Spur Gear 10 teeth (16)-dup (Autodesk Fusion 360 design; units mm, degrees)
description: Spur Gear; Module: 1.27; Num Teeth: 10; Pressure Angle: 20.0; Backlash: 0.00 mm
part number: 2026-06-06-03-03-36-066
Autodesk Fusion 360 part; units mm, degrees
(part 1 of 2)
sketch "Base Circle" plane through (0, 0, 0) normal (0, 0, 1) x (1, 0, 0)
  circle A0 centre (0, 0) radius 4.8806
  circle A1 centre (0, 0) radius 2.5
extrude "Extrude1" add sketch "Base Circle" along normal blind 1
sketch "Gear Tooth" plane through (0, 0, 0) normal (0, 0, 1) x (1, 0, 0)
  spline S0 degree 5 poles (5.879, -1.0212) (5.8838, -1.022) (5.8935, -1.0235) (5.908, -1.0253) (5.9275, -1.0267) (5.952, -1.0272) (5.9766, -1.0267) (6.0013, -1.0257) (6.026, -1.0244) (6.0508, -1.0228) (6.0756, -1.021) (6.1004, -1.0189) (6.1253, -1.0165) (6.1502, -1.0135) (6.1752, -1.0101) (6.2001, -1.0063) (6.2251, -1.002) (6.2502, -0.9975) (6.2752, -0.9927) (6.3003, -0.9876) (6.3253, -0.9823) (6.3504, -0.9767) (6.3755, -0.9708) (6.4006, -0.9646) (6.4257, -0.9581) (6.4508, -0.9513) (6.4759, -0.9442) (6.501, -0.9369) (6.5261, -0.9293) (6.5512, -0.9215) (6.5763, -0.9134) (6.6014, -0.9051) (6.6265, -0.8965) (6.6516, -0.8877) (6.6767, -0.8786) (6.7018, -0.8693) (6.7268, -0.8598) (6.7519, -0.85) (6.7769, -0.84) (6.8019, -0.8297) (6.8269, -0.8193) (6.8519, -0.8086) (6.8768, -0.7977) (6.9017, -0.7865) (6.9267, -0.7752) (6.9515, -0.7636) (6.9764, -0.7518) (7.0012, -0.7398) (7.0261, -0.7275) (7.0508, -0.7151) (7.0756, -0.7025) (7.1003, -0.6896) (7.125, -0.6765) (7.1497, -0.6632) (7.1743, -0.6498) (7.1989, -0.6361) (7.2235, -0.6222) (7.248, -0.6081) (7.2725, -0.5938) (7.2969, -0.5793) (7.3213, -0.5646) (7.3457, -0.5497) (7.37, -0.5346) (7.3943, -0.5193) (7.4186, -0.5038) (7.4428, -0.4882) (7.4669, -0.4723) (7.491, -0.4562) (7.5151, -0.44) (7.5391, -0.4236) (7.5631, -0.4069) (7.5822, -0.3935) (7.5966, -0.3833) (7.6061, -0.3765) (7.6109, -0.373) knots 0 0 0 0 0 0 0.01428571 0.02857143 0.04285714 0.05714286 0.07142857 0.08571429 0.1 0.11428571 0.12857143 0.14285714 0.15714286 0.17142857 0.18571429 0.2 0.21428571 0.22857143 0.24285714 0.25714286 0.27142857 0.28571429 0.3 0.31428571 0.32857143 0.34285714 0.35714286 0.37142857 0.38571429 0.4 0.41428571 0.42857143 0.44285714 0.45714286 0.47142857 0.48571429 0.5 0.51428571 0.52857143 0.54285714 0.55714286 0.57142857 0.58571429 0.6 0.61428571 0.62857143 0.64285714 0.65714286 0.67142857 0.68571429 0.7 0.71428571 0.72857143 0.74285714 0.75714286 0.77142857 0.78571429 0.8 0.81428571 0.82857143 0.84285714 0.85714286 0.87142857 0.88571429 0.9 0.91428571 0.92857143 0.94285714 0.95714286 0.97142857 0.98571429 1 1 1 1 1 1
  spline S1 degree 5 poles (5.879, 1.0212) (5.8838, 1.022) (5.8935, 1.0235) (5.908, 1.0253) (5.9275, 1.0267) (5.952, 1.0272) (5.9766, 1.0267) (6.0013, 1.0257) (6.026, 1.0244) (6.0508, 1.0228) (6.0756, 1.021) (6.1004, 1.0189) (6.1253, 1.0165) (6.1502, 1.0135) (6.1752, 1.0101) (6.2001, 1.0063) (6.2251, 1.002) (6.2502, 0.9975) (6.2752, 0.9927) (6.3003, 0.9876) (6.3253, 0.9823) (6.3504, 0.9767) (6.3755, 0.9708) (6.4006, 0.9646) (6.4257, 0.9581) (6.4508, 0.9513) (6.4759, 0.9442) (6.501, 0.9369) (6.5261, 0.9293) (6.5512, 0.9215) (6.5763, 0.9134) (6.6014, 0.9051) (6.6265, 0.8965) (6.6516, 0.8877) (6.6767, 0.8786) (6.7018, 0.8693) (6.7268, 0.8598) (6.7519, 0.85) (6.7769, 0.84) (6.8019, 0.8297) (6.8269, 0.8193) (6.8519, 0.8086) (6.8768, 0.7977) (6.9017, 0.7865) (6.9267, 0.7752) (6.9515, 0.7636) (6.9764, 0.7518) (7.0012, 0.7398) (7.0261, 0.7275) (7.0508, 0.7151) (7.0756, 0.7025) (7.1003, 0.6896) (7.125, 0.6765) (7.1497, 0.6632) (7.1743, 0.6498) (7.1989, 0.6361) (7.2235, 0.6222) (7.248, 0.6081) (7.2725, 0.5938) (7.2969, 0.5793) (7.3213, 0.5646) (7.3457, 0.5497) (7.37, 0.5346) (7.3943, 0.5193) (7.4186, 0.5038) (7.4428, 0.4882) (7.4669, 0.4723) (7.491, 0.4562) (7.5151, 0.44) (7.5391, 0.4236) (7.5631, 0.4069) (7.5822, 0.3935) (7.5966, 0.3833) (7.6061, 0.3765) (7.6109, 0.373) knots 0 0 0 0 0 0 0.01428571 0.02857143 0.04285714 0.05714286 0.07142857 0.08571429 0.1 0.11428571 0.12857143 0.14285714 0.15714286 0.17142857 0.18571429 0.2 0.21428571 0.22857143 0.24285714 0.25714286 0.27142857 0.28571429 0.3 0.31428571 0.32857143 0.34285714 0.35714286 0.37142857 0.38571429 0.4 0.41428571 0.42857143 0.44285714 0.45714286 0.47142857 0.48571429 0.5 0.51428571 0.52857143 0.54285714 0.55714286 0.57142857 0.58571429 0.6 0.61428571 0.62857143 0.64285714 0.65714286 0.67142857 0.68571429 0.7 0.71428571 0.72857143 0.74285714 0.75714286 0.77142857 0.78571429 0.8 0.81428571 0.82857143 0.84285714 0.85714286 0.87142857 0.88571429 0.9 0.91428571 0.92857143 0.94285714 0.95714286 0.97142857 0.98571429 1 1 1 1 1 1
  arc A0 (7.6109, -0.373) -> (7.6109, 0.373) centre (0, 0) ccw
  line L0 (4.7988, -0.8335) -> (5.879, -1.0212)
  line L1 (4.7988, 0.8335) -> (5.879, 1.0212)
  line L2 (4.7988, -0.8335) -> (4.7988, 0.8335)
  point P0 (5.998, -1.0258)
  point P1 (6.1192, -1.017)
  point P2 (6.2418, -0.999)
  point P3 (6.3654, -0.9731)
  point P4 (6.4896, -0.9402)
  point P5 (6.6144, -0.9006)
  point P6 (6.7395, -0.8548)
  point P7 (6.8648, -0.8029)
  point P8 (6.9901, -0.7452)
  point P9 (7.1151, -0.6817)
  point P10 (7.2399, -0.6127)
  point P11 (7.3642, -0.5382)
  point P12 (7.4879, -0.4583)
  point P13 (5.998, 1.0258)
  point P14 (6.1192, 1.017)
  point P15 (6.2418, 0.999)
  point P16 (6.3654, 0.9731)
  point P17 (6.4896, 0.9402)
  point P18 (6.6144, 0.9006)
  point P19 (6.7395, 0.8548)
  point P20 (6.8648, 0.8029)
  point P21 (6.9901, 0.7452)
  point P22 (7.1151, 0.6817)
  point P23 (7.2399, 0.6127)
  point P24 (7.3642, 0.5382)
  point P25 (7.4879, 0.4583)
extrude "Extrude2" add sketch "Gear Tooth" along normal blind 1
fillet "Fillet1" radius 0.2 2 edges at (4.8086, -0.8353, 0.5) (4.8086, 0.8353, 0.5)
pattern_circular "C-Pattern1" count 10 over 360 about axis through (0, 0, 0) along (0, 0, 1) of "Extrude2", "Fillet1"
sketch "Diametrial Pitch Circle" plane through (0, 0, 0) normal (0, 0, 1) x (1, 0, 0)
  circle A0 centre (0, 0) radius 6.35 construction
extrude "Extrude3" add 1 faces at (4.0508, 0, 0) along direction (0, 0, -1) blind 2
extrude "Extrude4" add 1 faces at (4.0508, 0, 1) along direction (0, 0, 1) blind 3
sketch "Sketch4" plane through (0, 0, 4) normal (0, 0, 1) x (1, 0, 0)
  arc A0 (4.4625, -1.9766) -> (4.772, -1.0239) centre (0, 0) ccw
  arc A1 (5.0018, -0.8688) -> (4.772, -1.0239) centre (4.9675, -1.0659) ccw
  line L0 (5.0018, -0.8688) -> (5.879, -1.0212)
  spline S0 degree 5 poles (5.879, -1.0212) (5.8838, -1.022) (5.8935, -1.0235) (5.908, -1.0253) (5.9275, -1.0267) (5.952, -1.0272) (5.9766, -1.0267) (6.0013, -1.0257) (6.026, -1.0244) (6.0508, -1.0228) (6.0756, -1.021) (6.1004, -1.0189) (6.1253, -1.0165) (6.1502, -1.0135) (6.1752, -1.0101) (6.2001, -1.0063) (6.2251, -1.002) (6.2502, -0.9975) (6.2752, -0.9927) (6.3003, -0.9876) (6.3253, -0.9823) (6.3504, -0.9767) (6.3755, -0.9708) (6.4006, -0.9646) (6.4257, -0.9581) (6.4508, -0.9513) (6.4759, -0.9442) (6.501, -0.9369) (6.5261, -0.9293) (6.5512, -0.9215) (6.5763, -0.9134) (6.6014, -0.9051) (6.6265, -0.8965) (6.6516, -0.8877) (6.6767, -0.8786) (6.7018, -0.8693) (6.7268, -0.8598) (6.7519, -0.85) (6.7769, -0.84) (6.8019, -0.8297) (6.8269, -0.8193) (6.8519, -0.8086) (6.8768, -0.7977) (6.9017, -0.7865) (6.9267, -0.7752) (6.9515, -0.7636) (6.9764, -0.7518) (7.0012, -0.7398) (7.0261, -0.7275) (7.0508, -0.7151) (7.0756, -0.7025) (7.1003, -0.6896) (7.125, -0.6765) (7.1497, -0.6632) (7.1743, -0.6498) (7.1989, -0.6361) (7.2235, -0.6222) (7.248, -0.6081) (7.2725, -0.5938) (7.2969, -0.5793) (7.3213, -0.5646) (7.3457, -0.5497) (7.37, -0.5346) (7.3943, -0.5193) (7.4186, -0.5038) (7.4428, -0.4882) (7.4669, -0.4723) (7.491, -0.4562) (7.5151, -0.44) (7.5391, -0.4236) (7.5631, -0.4069) (7.5822, -0.3935) (7.5966, -0.3833) (7.6061, -0.3765) (7.6109, -0.373) knots 0 0 0 0 0 0 0.01428571 0.02857143 0.04285714 0.05714286 0.07142857 0.08571429 0.1 0.11428571 0.12857143 0.14285714 0.15714286 0.17142857 0.18571429 0.2 0.21428571 0.22857143 0.24285714 0.25714286 0.27142857 0.28571429 0.3 0.31428571 0.32857143 0.34285714 0.35714286 0.37142857 0.38571429 0.4 0.41428571 0.42857143 0.44285714 0.45714286 0.47142857 0.48571429 0.5 0.51428571 0.52857143 0.54285714 0.55714286 0.57142857 0.58571429 0.6 0.61428571 0.62857143 0.64285714 0.65714286 0.67142857 0.68571429 0.7 0.71428571 0.72857143 0.74285714 0.75714286 0.77142857 0.78571429 0.8 0.81428571 0.82857143 0.84285714 0.85714286 0.87142857 0.88571429 0.9 0.91428571 0.92857143 0.94285714 0.95714286 0.97142857 0.98571429 1 1 1 1 1 1
  arc A2 (7.6109, -0.373) -> (7.6109, 0.373) centre (0, 0) ccw
  spline S1 degree 5 poles (7.6109, 0.373) (7.6061, 0.3765) (7.5966, 0.3833) (7.5822, 0.3935) (7.5631, 0.4069) (7.5391, 0.4236) (7.5151, 0.44) (7.491, 0.4562) (7.4669, 0.4723) (7.4428, 0.4882) (7.4186, 0.5038) (7.3943, 0.5193) (7.37, 0.5346) (7.3457, 0.5497) (7.3213, 0.5646) (7.2969, 0.5793) (7.2725, 0.5938) (7.248, 0.6081) (7.2235, 0.6222) (7.1989, 0.6361) (7.1743, 0.6498) (7.1497, 0.6632) (7.125, 0.6765) (7.1003, 0.6896) (7.0756, 0.7025) (7.0508, 0.7151) (7.0261, 0.7275) (7.0012, 0.7398) (6.9764, 0.7518) (6.9515, 0.7636) (6.9267, 0.7752) (6.9017, 0.7865) (6.8768, 0.7977) (6.8519, 0.8086) (6.8269, 0.8193) (6.8019, 0.8297) (6.7769, 0.84) (6.7519, 0.85) (6.7268, 0.8598) (6.7018, 0.8693) (6.6767, 0.8786) (6.6516, 0.8877) (6.6265, 0.8965) (6.6014, 0.9051) (6.5763, 0.9134) (6.5512, 0.9215) (6.5261, 0.9293) (6.501, 0.9369) (6.4759, 0.9442) (6.4508, 0.9513) (6.4257, 0.9581) (6.4006, 0.9646) (6.3755, 0.9708) (6.3504, 0.9767) (6.3253, 0.9823) (6.3003, 0.9876) (6.2752, 0.9927) (6.2502, 0.9975) (6.2251, 1.002) (6.2001, 1.0063) (6.1752, 1.0101) (6.1502, 1.0135) (6.1253, 1.0165) (6.1004, 1.0189) (6.0756, 1.021) (6.0508, 1.0228) (6.026, 1.0244) (6.0013, 1.0257) (5.9766, 1.0267) (5.952, 1.0272) (5.9275, 1.0267) (5.908, 1.0253) (5.8935, 1.0235) (5.8838, 1.022) (5.879, 1.0212) knots -1 -1 -1 -1 -1 -1 -0.98571429 -0.97142857 -0.95714286 -0.94285714 -0.92857143 -0.91428571 -0.9 -0.88571429 -0.87142857 -0.85714286 -0.84285714 -0.82857143 -0.81428571 -0.8 -0.78571429 -0.77142857 -0.75714286 -0.74285714 -0.72857143 -0.71428571 -0.7 -0.68571429 -0.67142857 -0.65714286 -0.64285714 -0.62857143 -0.61428571 -0.6 -0.58571429 -0.57142857 -0.55714286 -0.54285714 -0.52857143 -0.51428571 -0.5 -0.48571429 -0.47142857 -0.45714286 -0.44285714 -0.42857143 -0.41428571 -0.4 -0.38571429 -0.37142857 -0.35714286 -0.34285714 -0.32857143 -0.31428571 -0.3 -0.28571429 -0.27142857 -0.25714286 -0.24285714 -0.22857143 -0.21428571 -0.2 -0.18571429 -0.17142857 -0.15714286 -0.14285714 -0.12857143 -0.11428571 -0.1 -0.08571429 -0.07142857 -0.05714286 -0.04285714 -0.02857143 -0.01428571 0 0 0 0 0 0
  line L1 (5.879, 1.0212) -> (5.0018, 0.8688)
  arc A3 (4.772, 1.0239) -> (5.0018, 0.8688) centre (4.9675, 1.0659) ccw
  arc A4 (4.772, 1.0239) -> (4.4625, 1.9766) centre (0, 0) ccw
  arc A5 (4.5572, 2.2371) -> (4.4625, 1.9766) centre (4.6453, 2.0576) ccw
  line L2 (4.5572, 2.2371) -> (5.3565, 2.6294)
  spline S2 degree 5 poles (5.3565, 2.6294) (5.3609, 2.6316) (5.3696, 2.6361) (5.3824, 2.6432) (5.3989, 2.6535) (5.419, 2.6675) (5.4387, 2.6823) (5.458, 2.6976) (5.4773, 2.7133) (5.4964, 2.7291) (5.5154, 2.7451) (5.5343, 2.7614) (5.5529, 2.778) (5.5713, 2.7951) (5.5895, 2.8125) (5.6075, 2.8303) (5.6252, 2.8484) (5.6428, 2.8668) (5.6602, 2.8854) (5.6775, 2.9042) (5.6947, 2.9233) (5.7117, 2.9425) (5.7285, 2.9621) (5.7451, 2.9818) (5.7616, 3.0018) (5.7779, 3.0221) (5.7941, 3.0426) (5.8101, 3.0633) (5.826, 3.0842) (5.8417, 3.1052) (5.8572, 3.1265) (5.8727, 3.148) (5.8879, 3.1697) (5.903, 3.1916) (5.918, 3.2137) (5.9328, 3.2359) (5.9475, 3.2584) (5.962, 3.281) (5.9763, 3.3038) (5.9905, 3.3268) (6.0046, 3.3499) (6.0185, 3.3733) (6.0323, 3.3968) (6.0459, 3.4204) (6.0594, 3.4443) (6.0727, 3.4683) (6.0859, 3.4924) (6.099, 3.5167) (6.1118, 3.5412) (6.1246, 3.5658) (6.1372, 3.5906) (6.1496, 3.6156) (6.1619, 3.6407) (6.1741, 3.6659) (6.1861, 3.6913) (6.1979, 3.7168) (6.2096, 3.7425) (6.2212, 3.7683) (6.2326, 3.7943) (6.2438, 3.8204) (6.255, 3.8466) (6.2659, 3.873) (6.2767, 3.8995) (6.2874, 3.9261) (6.2979, 3.9529) (6.3083, 3.9798) (6.3185, 4.0069) (6.3286, 4.034) (6.3385, 4.0613) (6.3482, 4.0887) (6.3579, 4.1163) (6.3654, 4.1384) (6.371, 4.1551) (6.3747, 4.1662) (6.3766, 4.1718) knots 0 0 0 0 0 0 0.01428571 0.02857143 0.04285714 0.05714286 0.07142857 0.08571429 0.1 0.11428571 0.12857143 0.14285714 0.15714286 0.17142857 0.18571429 0.2 0.21428571 0.22857143 0.24285714 0.25714286 0.27142857 0.28571429 0.3 0.31428571 0.32857143 0.34285714 0.35714286 0.37142857 0.38571429 0.4 0.41428571 0.42857143 0.44285714 0.45714286 0.47142857 0.48571429 0.5 0.51428571 0.52857143 0.54285714 0.55714286 0.57142857 0.58571429 0.6 0.61428571 0.62857143 0.64285714 0.65714286 0.67142857 0.68571429 0.7 0.71428571 0.72857143 0.74285714 0.75714286 0.77142857 0.78571429 0.8 0.81428571 0.82857143 0.84285714 0.85714286 0.87142857 0.88571429 0.9 0.91428571 0.92857143 0.94285714 0.95714286 0.97142857 0.98571429 1 1 1 1 1 1
  arc A6 (6.3766, 4.1718) -> (5.938, 4.7754) centre (0, 0) ccw
  spline S3 degree 5 poles (5.938, 4.7754) (5.9322, 4.7753) (5.9204, 4.7752) (5.9029, 4.775) (5.8795, 4.7747) (5.8503, 4.774) (5.8212, 4.7732) (5.7922, 4.7722) (5.7633, 4.7711) (5.7344, 4.7697) (5.7056, 4.7682) (5.6769, 4.7664) (5.6483, 4.7645) (5.6197, 4.7624) (5.5912, 4.7602) (5.5628, 4.7577) (5.5345, 4.755) (5.5063, 4.7522) (5.4782, 4.7492) (5.4502, 4.746) (5.4222, 4.7426) (5.3944, 4.7391) (5.3666, 4.7353) (5.3389, 4.7314) (5.3114, 4.7272) (5.2839, 4.7229) (5.2566, 4.7184) (5.2293, 4.7137) (5.2021, 4.7088) (5.1751, 4.7038) (5.1481, 4.6985) (5.1213, 4.6931) (5.0946, 4.6874) (5.068, 4.6816) (5.0415, 4.6755) (5.0151, 4.6693) (4.9889, 4.6629) (4.9628, 4.6563) (4.9368, 4.6495) (4.9109, 4.6425) (4.8851, 4.6353) (4.8595, 4.6279) (4.834, 4.6203) (4.8087, 4.6124) (4.7835, 4.6044) (4.7584, 4.5962) (4.7335, 4.5878) (4.7088, 4.5791) (4.6841, 4.5703) (4.6597, 4.5613) (4.6354, 4.552) (4.6112, 4.5425) (4.5873, 4.5328) (4.5635, 4.5228) (4.5399, 4.5126) (4.5165, 4.5022) (4.4933, 4.4916) (4.4702, 4.4807) (4.4473, 4.4697) (4.4246, 4.4584) (4.4021, 4.4468) (4.3799, 4.4349) (4.358, 4.4227) (4.3364, 4.4101) (4.3151, 4.3972) (4.294, 4.384) (4.273, 4.3707) (4.2522, 4.3573) (4.2317, 4.3436) (4.2115, 4.3295) (4.192, 4.3147) (4.177, 4.3021) (4.1663, 4.2922) (4.1594, 4.2853) (4.156, 4.2818) knots -1 -1 -1 -1 -1 -1 -0.98571429 -0.97142857 -0.95714286 -0.94285714 -0.92857143 -0.91428571 -0.9 -0.88571429 -0.87142857 -0.85714286 -0.84285714 -0.82857143 -0.81428571 -0.8 -0.78571429 -0.77142857 -0.75714286 -0.74285714 -0.72857143 -0.71428571 -0.7 -0.68571429 -0.67142857 -0.65714286 -0.64285714 -0.62857143 -0.61428571 -0.6 -0.58571429 -0.57142857 -0.55714286 -0.54285714 -0.52857143 -0.51428571 -0.5 -0.48571429 -0.47142857 -0.45714286 -0.44285714 -0.42857143 -0.41428571 -0.4 -0.38571429 -0.37142857 -0.35714286 -0.34285714 -0.32857143 -0.31428571 -0.3 -0.28571429 -0.27142857 -0.25714286 -0.24285714 -0.22857143 -0.21428571 -0.2 -0.18571429 -0.17142857 -0.15714286 -0.14285714 -0.12857143 -0.11428571 -0.1 -0.08571429 -0.07142857 -0.05714286 -0.04285714 -0.02857143 -0.01428571 0 0 0 0 0 0
  line L3 (4.156, 4.2818) -> (3.5358, 3.6429)
  arc A7 (3.2588, 3.6333) -> (3.5358, 3.6429) centre (3.3923, 3.7821) ccw
  arc A8 (3.2588, 3.6333) -> (2.4484, 4.222) centre (0, 0) ccw
  arc A9 (2.3719, 4.4885) -> (2.4484, 4.222) centre (2.5487, 4.3951) ccw
  line L4 (2.3719, 4.4885) -> (2.7879, 5.2757)
  spline S4 degree 5 poles (2.7879, 5.2757) (2.7902, 5.28) (2.7946, 5.2888) (2.8008, 5.302) (2.8082, 5.3201) (2.8162, 5.3433) (2.8234, 5.3668) (2.83, 5.3906) (2.8364, 5.4145) (2.8426, 5.4386) (2.8485, 5.4627) (2.8542, 5.487) (2.8595, 5.5114) (2.8644, 5.536) (2.8689, 5.5608) (2.8729, 5.5857) (2.8767, 5.6108) (2.8801, 5.636) (2.8832, 5.6613) (2.8862, 5.6867) (2.8888, 5.7122) (2.8912, 5.7378) (2.8934, 5.7635) (2.8952, 5.7893) (2.8968, 5.8151) (2.8981, 5.8411) (2.8991, 5.8672) (2.8999, 5.8933) (2.9005, 5.9196) (2.9008, 5.9459) (2.9009, 5.9722) (2.9007, 5.9987) (2.9003, 6.0252) (2.8997, 6.0518) (2.8988, 6.0784) (2.8977, 6.1051) (2.8964, 6.1319) (2.8948, 6.1587) (2.893, 6.1856) (2.891, 6.2126) (2.8888, 6.2396) (2.8863, 6.2666) (2.8837, 6.2937) (2.8808, 6.3209) (2.8777, 6.3481) (2.8744, 6.3753) (2.8708, 6.4026) (2.8671, 6.43) (2.8631, 6.4574) (2.8589, 6.4848) (2.8546, 6.5122) (2.85, 6.5397) (2.8452, 6.5672) (2.8402, 6.5948) (2.8349, 6.6224) (2.8295, 6.65) (2.8239, 6.6777) (2.8181, 6.7053) (2.8121, 6.7331) (2.8058, 6.7608) (2.7994, 6.7885) (2.7928, 6.8163) (2.7859, 6.8441) (2.7789, 6.872) (2.7717, 6.8998) (2.7642, 6.9277) (2.7566, 6.9555) (2.7488, 6.9834) (2.7408, 7.0113) (2.7325, 7.0392) (2.7241, 7.0672) (2.7172, 7.0895) (2.712, 7.1063) (2.7085, 7.1175) (2.7067, 7.1231) knots 0 0 0 0 0 0 0.01428571 0.02857143 0.04285714 0.05714286 0.07142857 0.08571429 0.1 0.11428571 0.12857143 0.14285714 0.15714286 0.17142857 0.18571429 0.2 0.21428571 0.22857143 0.24285714 0.25714286 0.27142857 0.28571429 0.3 0.31428571 0.32857143 0.34285714 0.35714286 0.37142857 0.38571429 0.4 0.41428571 0.42857143 0.44285714 0.45714286 0.47142857 0.48571429 0.5 0.51428571 0.52857143 0.54285714 0.55714286 0.57142857 0.58571429 0.6 0.61428571 0.62857143 0.64285714 0.65714286 0.67142857 0.68571429 0.7 0.71428571 0.72857143 0.74285714 0.75714286 0.77142857 0.78571429 0.8 0.81428571 0.82857143 0.84285714 0.85714286 0.87142857 0.88571429 0.9 0.91428571 0.92857143 0.94285714 0.95714286 0.97142857 0.98571429 1 1 1 1 1 1
  arc A10 (2.7067, 7.1231) -> (1.9971, 7.3536) centre (0, 0) ccw
  spline S5 degree 5 poles (1.9971, 7.3536) (1.9924, 7.3502) (1.9829, 7.3432) (1.9688, 7.3327) (1.9501, 7.3187) (1.9269, 7.301) (1.9038, 7.2833) (1.8809, 7.2654) (1.8582, 7.2474) (1.8357, 7.2294) (1.8133, 7.2112) (1.7911, 7.1929) (1.769, 7.1745) (1.7471, 7.1561) (1.7255, 7.1375) (1.7039, 7.1188) (1.6826, 7.1) (1.6614, 7.0812) (1.6404, 7.0622) (1.6196, 7.0431) (1.599, 7.024) (1.5786, 7.0047) (1.5583, 6.9854) (1.5383, 6.9659) (1.5184, 6.9464) (1.4987, 6.9267) (1.4792, 6.907) (1.4599, 6.8872) (1.4408, 6.8673) (1.4219, 6.8473) (1.4032, 6.8272) (1.3847, 6.807) (1.3664, 6.7867) (1.3483, 6.7664) (1.3305, 6.7459) (1.3128, 6.7254) (1.2953, 6.7048) (1.2781, 6.6841) (1.261, 6.6633) (1.2442, 6.6424) (1.2276, 6.6214) (1.2112, 6.6004) (1.1951, 6.5792) (1.1792, 6.558) (1.1635, 6.5367) (1.1481, 6.5153) (1.1329, 6.4939) (1.1179, 6.4723) (1.1032, 6.4507) (1.0887, 6.429) (1.0745, 6.4072) (1.0605, 6.3854) (1.0469, 6.3634) (1.0335, 6.3414) (1.0204, 6.3193) (1.0076, 6.2971) (0.995, 6.2748) (0.9827, 6.2525) (0.9707, 6.2301) (0.9589, 6.2076) (0.9476, 6.1851) (0.9366, 6.1624) (0.9261, 6.1396) (0.9161, 6.1167) (0.9064, 6.0937) (0.897, 6.0707) (0.8879, 6.0476) (0.879, 6.0245) (0.8704, 6.0014) (0.8623, 5.9781) (0.8552, 5.9547) (0.8506, 5.9357) (0.8478, 5.9213) (0.8462, 5.9117) (0.8455, 5.9068) knots -1 -1 -1 -1 -1 -1 -0.98571429 -0.97142857 -0.95714286 -0.94285714 -0.92857143 -0.91428571 -0.9 -0.88571429 -0.87142857 -0.85714286 -0.84285714 -0.82857143 -0.81428571 -0.8 -0.78571429 -0.77142857 -0.75714286 -0.74285714 -0.72857143 -0.71428571 -0.7 -0.68571429 -0.67142857 -0.65714286 -0.64285714 -0.62857143 -0.61428571 -0.6 -0.58571429 -0.57142857 -0.55714286 -0.54285714 -0.52857143 -0.51428571 -0.5 -0.48571429 -0.47142857 -0.45714286 -0.44285714 -0.42857143 -0.41428571 -0.4 -0.38571429 -0.37142857 -0.35714286 -0.34285714 -0.32857143 -0.31428571 -0.3 -0.28571429 -0.27142857 -0.25714286 -0.24285714 -0.22857143 -0.21428571 -0.2 -0.18571429 -0.17142857 -0.15714286 -0.14285714 -0.12857143 -0.11428571 -0.1 -0.08571429 -0.07142857 -0.05714286 -0.04285714 -0.02857143 -0.01428571 0 0 0 0 0 0
  line L5 (0.8455, 5.9068) -> (0.7193, 5.0254)
  arc A11 (0.5008, 4.8548) -> (0.7193, 5.0254) centre (0.5214, 5.0538) ccw
  arc A12 (0.5008, 4.8548) -> (-0.5008, 4.8548) centre (0, 0) ccw
  arc A13 (-0.7193, 5.0254) -> (-0.5008, 4.8548) centre (-0.5214, 5.0538) ccw
  line L6 (-0.7193, 5.0254) -> (-0.8455, 5.9068)
  spline S6 degree 5 poles (-0.8455, 5.9068) (-0.8462, 5.9117) (-0.8478, 5.9213) (-0.8506, 5.9357) (-0.8552, 5.9547) (-0.8623, 5.9781) (-0.8704, 6.0014) (-0.879, 6.0245) (-0.8879, 6.0476) (-0.897, 6.0707) (-0.9064, 6.0937) (-0.9161, 6.1167) (-0.9261, 6.1396) (-0.9366, 6.1624) (-0.9476, 6.1851) (-0.9589, 6.2076) (-0.9707, 6.2301) (-0.9827, 6.2525) (-0.995, 6.2748) (-1.0076, 6.2971) (-1.0204, 6.3193) (-1.0335, 6.3414) (-1.0469, 6.3634) (-1.0605, 6.3854) (-1.0745, 6.4072) (-1.0887, 6.429) (-1.1032, 6.4507) (-1.1179, 6.4723) (-1.1329, 6.4939) (-1.1481, 6.5153) (-1.1635, 6.5367) (-1.1792, 6.558) (-1.1951, 6.5792) (-1.2112, 6.6004) (-1.2276, 6.6214) (-1.2442, 6.6424) (-1.261, 6.6633) (-1.2781, 6.6841) (-1.2953, 6.7048) (-1.3128, 6.7254) (-1.3305, 6.7459) (-1.3483, 6.7664) (-1.3664, 6.7867) (-1.3847, 6.807) (-1.4032, 6.8272) (-1.4219, 6.8473) (-1.4408, 6.8673) (-1.4599, 6.8872) (-1.4792, 6.907) (-1.4987, 6.9267) (-1.5184, 6.9464) (-1.5383, 6.9659) (-1.5583, 6.9854) (-1.5786, 7.0047) (-1.599, 7.024) (-1.6196, 7.0431) (-1.6404, 7.0622) (-1.6614, 7.0812) (-1.6826, 7.1) (-1.7039, 7.1188) (-1.7255, 7.1375) (-1.7471, 7.1561) (-1.769, 7.1745) (-1.7911, 7.1929) (-1.8133, 7.2112) (-1.8357, 7.2294) (-1.8582, 7.2474) (-1.8809, 7.2654) (-1.9038, 7.2833) (-1.9269, 7.301) (-1.9501, 7.3187) (-1.9688, 7.3327) (-1.9829, 7.3432) (-1.9924, 7.3502) (-1.9971, 7.3536) knots 0 0 0 0 0 0 0.01428571 0.02857143 0.04285714 0.05714286 0.07142857 0.08571429 0.1 0.11428571 0.12857143 0.14285714 0.15714286 0.17142857 0.18571429 0.2 0.21428571 0.22857143 0.24285714 0.25714286 0.27142857 0.28571429 0.3 0.31428571 0.32857143 0.34285714 0.35714286 0.37142857 0.38571429 0.4 0.41428571 0.42857143 0.44285714 0.45714286 0.47142857 0.48571429 0.5 0.51428571 0.52857143 0.54285714 0.55714286 0.57142857 0.58571429 0.6 0.61428571 0.62857143 0.64285714 0.65714286 0.67142857 0.68571429 0.7 0.71428571 0.72857143 0.74285714 0.75714286 0.77142857 0.78571429 0.8 0.81428571 0.82857143 0.84285714 0.85714286 0.87142857 0.88571429 0.9 0.91428571 0.92857143 0.94285714 0.95714286 0.97142857 0.98571429 1 1 1 1 1 1
  arc A14 (-1.9971, 7.3536) -> (-2.7067, 7.1231) centre (0, 0) ccw
  spline S7 degree 5 poles (-2.7067, 7.1231) (-2.7085, 7.1175) (-2.712, 7.1063) (-2.7172, 7.0895) (-2.7241, 7.0672) (-2.7325, 7.0392) (-2.7408, 7.0113) (-2.7488, 6.9834) (-2.7566, 6.9555) (-2.7642, 6.9277) (-2.7717, 6.8998) (-2.7789, 6.872) (-2.7859, 6.8441) (-2.7928, 6.8163) (-2.7994, 6.7885) (-2.8058, 6.7608) (-2.8121, 6.7331) (-2.8181, 6.7053) (-2.8239, 6.6777) (-2.8295, 6.65) (-2.8349, 6.6224) (-2.8402, 6.5948) (-2.8452, 6.5672) (-2.85, 6.5397) (-2.8546, 6.5122) (-2.8589, 6.4848) (-2.8631, 6.4574) (-2.8671, 6.43) (-2.8708, 6.4026) (-2.8744, 6.3753) (-2.8777, 6.3481) (-2.8808, 6.3209) (-2.8837, 6.2937) (-2.8863, 6.2666) (-2.8888, 6.2396) (-2.891, 6.2126) (-2.893, 6.1856) (-2.8948, 6.1587) (-2.8964, 6.1319) (-2.8977, 6.1051) (-2.8988, 6.0784) (-2.8997, 6.0518) (-2.9003, 6.0252) (-2.9007, 5.9987) (-2.9009, 5.9722) (-2.9008, 5.9459) (-2.9005, 5.9196) (-2.8999, 5.8933) (-2.8991, 5.8672) (-2.8981, 5.8411) (-2.8968, 5.8151) (-2.8952, 5.7893) (-2.8934, 5.7635) (-2.8912, 5.7378) (-2.8888, 5.7122) (-2.8862, 5.6867) (-2.8832, 5.6613) (-2.8801, 5.636) (-2.8767, 5.6108) (-2.8729, 5.5857) (-2.8689, 5.5608) (-2.8644, 5.536) (-2.8595, 5.5114) (-2.8542, 5.487) (-2.8485, 5.4627) (-2.8426, 5.4386) (-2.8364, 5.4145) (-2.83, 5.3906) (-2.8234, 5.3668) (-2.8162, 5.3433) (-2.8082, 5.3201) (-2.8008, 5.302) (-2.7946, 5.2888) (-2.7902, 5.28) (-2.7879, 5.2757) knots -1 -1 -1 -1 -1 -1 -0.98571429 -0.97142857 -0.95714286 -0.94285714 -0.92857143 -0.91428571 -0.9 -0.88571429 -0.87142857 -0.85714286 -0.84285714 -0.82857143 -0.81428571 -0.8 -0.78571429 -0.77142857 -0.75714286 -0.74285714 -0.72857143 -0.71428571 -0.7 -0.68571429 -0.67142857 -0.65714286 -0.64285714 -0.62857143 -0.61428571 -0.6 -0.58571429 -0.57142857 -0.55714286 -0.54285714 -0.52857143 -0.51428571 -0.5 -0.48571429 -0.47142857 -0.45714286 -0.44285714 -0.42857143 -0.41428571 -0.4 -0.38571429 -0.37142857 -0.35714286 -0.34285714 -0.32857143 -0.31428571 -0.3 -0.28571429 -0.27142857 -0.25714286 -0.24285714 -0.22857143 -0.21428571 -0.2 -0.18571429 -0.17142857 -0.15714286 -0.14285714 -0.12857143 -0.11428571 -0.1 -0.08571429 -0.07142857 -0.05714286 -0.04285714 -0.02857143 -0.01428571 0 0 0 0 0 0
  line L7 (-2.7879, 5.2757) -> (-2.3719, 4.4885)
  arc A15 (-2.4484, 4.222) -> (-2.3719, 4.4885) centre (-2.5487, 4.3951) ccw
  arc A16 (-2.4484, 4.222) -> (-3.2588, 3.6333) centre (0, 0) ccw
  arc A17 (-3.5358, 3.6429) -> (-3.2588, 3.6333) centre (-3.3923, 3.7821) ccw
  line L8 (-3.5358, 3.6429) -> (-4.156, 4.2818)
  spline S8 degree 5 poles (-4.156, 4.2818) (-4.1594, 4.2853) (-4.1663, 4.2922) (-4.177, 4.3021) (-4.192, 4.3147) (-4.2115, 4.3295) (-4.2317, 4.3436) (-4.2522, 4.3573) (-4.273, 4.3707) (-4.294, 4.384) (-4.3151, 4.3972) (-4.3364, 4.4101) (-4.358, 4.4227) (-4.3799, 4.4349) (-4.4021, 4.4468) (-4.4246, 4.4584) (-4.4473, 4.4697) (-4.4702, 4.4807) (-4.4933, 4.4916) (-4.5165, 4.5022) (-4.5399, 4.5126) (-4.5635, 4.5228) (-4.5873, 4.5328) (-4.6112, 4.5425) (-4.6354, 4.552) (-4.6597, 4.5613) (-4.6841, 4.5703) (-4.7088, 4.5791) (-4.7335, 4.5878) (-4.7584, 4.5962) (-4.7835, 4.6044) (-4.8087, 4.6124) (-4.834, 4.6203) (-4.8595, 4.6279) (-4.8851, 4.6353) (-4.9109, 4.6425) (-4.9368, 4.6495) (-4.9628, 4.6563) (-4.9889, 4.6629) (-5.0151, 4.6693) (-5.0415, 4.6755) (-5.068, 4.6816) (-5.0946, 4.6874) (-5.1213, 4.6931) (-5.1481, 4.6985) (-5.1751, 4.7038) (-5.2021, 4.7088) (-5.2293, 4.7137) (-5.2566, 4.7184) (-5.2839, 4.7229) (-5.3114, 4.7272) (-5.3389, 4.7314) (-5.3666, 4.7353) (-5.3944, 4.7391) (-5.4222, 4.7426) (-5.4502, 4.746) (-5.4782, 4.7492) (-5.5063, 4.7522) (-5.5345, 4.755) (-5.5628, 4.7577) (-5.5912, 4.7602) (-5.6197, 4.7624) (-5.6483, 4.7645) (-5.6769, 4.7664) (-5.7056, 4.7682) (-5.7344, 4.7697) (-5.7633, 4.7711) (-5.7922, 4.7722) (-5.8212, 4.7732) (-5.8503, 4.774) (-5.8795, 4.7747) (-5.9029, 4.775) (-5.9204, 4.7752) (-5.9322, 4.7753) (-5.938, 4.7754) knots 0 0 0 0 0 0 0.01428571 0.02857143 0.04285714 0.05714286 0.07142857 0.08571429 0.1 0.11428571 0.12857143 0.14285714 0.15714286 0.17142857 0.18571429 0.2 0.21428571 0.22857143 0.24285714 0.25714286 0.27142857 0.28571429 0.3 0.31428571 0.32857143 0.34285714 0.35714286 0.37142857 0.38571429 0.4 0.41428571 0.42857143 0.44285714 0.45714286 0.47142857 0.48571429 0.5 0.51428571 0.52857143 0.54285714 0.55714286 0.57142857 0.58571429 0.6 0.61428571 0.62857143 0.64285714 0.65714286 0.67142857 0.68571429 0.7 0.71428571 0.72857143 0.74285714 0.75714286 0.77142857 0.78571429 0.8 0.81428571 0.82857143 0.84285714 0.85714286 0.87142857 0.88571429 0.9 0.91428571 0.92857143 0.94285714 0.95714286 0.97142857 0.98571429 1 1 1 1 1 1
  arc A18 (-5.938, 4.7754) -> (-6.3766, 4.1718) centre (0, 0) ccw
  spline S9 degree 5 poles (-6.3766, 4.1718) (-6.3747, 4.1662) (-6.371, 4.1551) (-6.3654, 4.1384) (-6.3579, 4.1163) (-6.3482, 4.0887) (-6.3385, 4.0613) (-6.3286, 4.034) (-6.3185, 4.0069) (-6.3083, 3.9798) (-6.2979, 3.9529) (-6.2874, 3.9261) (-6.2767, 3.8995) (-6.2659, 3.873) (-6.255, 3.8466) (-6.2438, 3.8204) (-6.2326, 3.7943) (-6.2212, 3.7683) (-6.2096, 3.7425) (-6.1979, 3.7168) (-6.1861, 3.6913) (-6.1741, 3.6659) (-6.1619, 3.6407) (-6.1496, 3.6156) (-6.1372, 3.5906) (-6.1246, 3.5658) (-6.1118, 3.5412) (-6.099, 3.5167) (-6.0859, 3.4924) (-6.0727, 3.4683) (-6.0594, 3.4443) (-6.0459, 3.4204) (-6.0323, 3.3968) (-6.0185, 3.3733) (-6.0046, 3.3499) (-5.9905, 3.3268) (-5.9763, 3.3038) (-5.962, 3.281) (-5.9475, 3.2584) (-5.9328, 3.2359) (-5.918, 3.2137) (-5.903, 3.1916) (-5.8879, 3.1697) (-5.8727, 3.148) (-5.8572, 3.1265) (-5.8417, 3.1052) (-5.826, 3.0842) (-5.8101, 3.0633) (-5.7941, 3.0426) (-5.7779, 3.0221) (-5.7616, 3.0018) (-5.7451, 2.9818) (-5.7285, 2.9621) (-5.7117, 2.9425) (-5.6947, 2.9233) (-5.6775, 2.9042) (-5.6602, 2.8854) (-5.6428, 2.8668) (-5.6252, 2.8484) (-5.6075, 2.8303) (-5.5895, 2.8125) (-5.5713, 2.7951) (-5.5529, 2.778) (-5.5343, 2.7614) (-5.5154, 2.7451) (-5.4964, 2.7291) (-5.4773, 2.7133) (-5.458, 2.6976) (-5.4387, 2.6823) (-5.419, 2.6675) (-5.3989, 2.6535) (-5.3824, 2.6432) (-5.3696, 2.6361) (-5.3609, 2.6316) (-5.3565, 2.6294) knots -1 -1 -1 -1 -1 -1 -0.98571429 -0.97142857 -0.95714286 -0.94285714 -0.92857143 -0.91428571 -0.9 -0.88571429 -0.87142857 -0.85714286 -0.84285714 -0.82857143 -0.81428571 -0.8 -0.78571429 -0.77142857 -0.75714286 -0.74285714 -0.72857143 -0.71428571 -0.7 -0.68571429 -0.67142857 -0.65714286 -0.64285714 -0.62857143 -0.61428571 -0.6 -0.58571429 -0.57142857 -0.55714286 -0.54285714 -0.52857143 -0.51428571 -0.5 -0.48571429 -0.47142857 -0.45714286 -0.44285714 -0.42857143 -0.41428571 -0.4 -0.38571429 -0.37142857 -0.35714286 -0.34285714 -0.32857143 -0.31428571 -0.3 -0.28571429 -0.27142857 -0.25714286 -0.24285714 -0.22857143 -0.21428571 -0.2 -0.18571429 -0.17142857 -0.15714286 -0.14285714 -0.12857143 -0.11428571 -0.1 -0.08571429 -0.07142857 -0.05714286 -0.04285714 -0.02857143 -0.01428571 0 0 0 0 0 0
  line L9 (-5.3565, 2.6294) -> (-4.5572, 2.2371)
  arc A19 (-4.4625, 1.9766) -> (-4.5572, 2.2371) centre (-4.6453, 2.0576) ccw
  arc A20 (-4.4625, 1.9766) -> (-4.772, 1.0239) centre (0, 0) ccw
  arc A21 (-5.0018, 0.8688) -> (-4.772, 1.0239) centre (-4.9675, 1.0659) ccw
  line L10 (-5.0018, 0.8688) -> (-5.879, 1.0212)
  spline S10 degree 5 poles (-5.879, 1.0212) (-5.8838, 1.022) (-5.8935, 1.0235) (-5.908, 1.0253) (-5.9275, 1.0267) (-5.952, 1.0272) (-5.9766, 1.0267) (-6.0013, 1.0257) (-6.026, 1.0244) (-6.0508, 1.0228) (-6.0756, 1.021) (-6.1004, 1.0189) (-6.1253, 1.0165) (-6.1502, 1.0135) (-6.1752, 1.0101) (-6.2001, 1.0063) (-6.2251, 1.002) (-6.2502, 0.9975) (-6.2752, 0.9927) (-6.3003, 0.9876) (-6.3253, 0.9823) (-6.3504, 0.9767) (-6.3755, 0.9708) (-6.4006, 0.9646) (-6.4257, 0.9581) (-6.4508, 0.9513) (-6.4759, 0.9442) (-6.501, 0.9369) (-6.5261, 0.9293) (-6.5512, 0.9215) (-6.5763, 0.9134) (-6.6014, 0.9051) (-6.6265, 0.8965) (-6.6516, 0.8877) (-6.6767, 0.8786) (-6.7018, 0.8693) (-6.7268, 0.8598) (-6.7519, 0.85) (-6.7769, 0.84) (-6.8019, 0.8297) (-6.8269, 0.8193) (-6.8519, 0.8086) (-6.8768, 0.7977) (-6.9017, 0.7865) (-6.9267, 0.7752) (-6.9515, 0.7636) (-6.9764, 0.7518) (-7.0012, 0.7398) (-7.0261, 0.7275) (-7.0508, 0.7151) (-7.0756, 0.7025) (-7.1003, 0.6896) (-7.125, 0.6765) (-7.1497, 0.6632) (-7.1743, 0.6498) (-7.1989, 0.6361) (-7.2235, 0.6222) (-7.248, 0.6081) (-7.2725, 0.5938) (-7.2969, 0.5793) (-7.3213, 0.5646) (-7.3457, 0.5497) (-7.37, 0.5346) (-7.3943, 0.5193) (-7.4186, 0.5038) (-7.4428, 0.4882) (-7.4669, 0.4723) (-7.491, 0.4562) (-7.5151, 0.44) (-7.5391, 0.4236) (-7.5631, 0.4069) (-7.5822, 0.3935) (-7.5966, 0.3833) (-7.6061, 0.3765) (-7.6109, 0.373) knots 0 0 0 0 0 0 0.01428571 0.02857143 0.04285714 0.05714286 0.07142857 0.08571429 0.1 0.11428571 0.12857143 0.14285714 0.15714286 0.17142857 0.18571429 0.2 0.21428571 0.22857143 0.24285714 0.25714286 0.27142857 0.28571429 0.3 0.31428571 0.32857143 0.34285714 0.35714286 0.37142857 0.38571429 0.4 0.41428571 0.42857143 0.44285714 0.45714286 0.47142857 0.48571429 0.5 0.51428571 0.52857143 0.54285714 0.55714286 0.57142857 0.58571429 0.6 0.61428571 0.62857143 0.64285714 0.65714286 0.67142857 0.68571429 0.7 0.71428571 0.72857143 0.74285714 0.75714286 0.77142857 0.78571429 0.8 0.81428571 0.82857143 0.84285714 0.85714286 0.87142857 0.88571429 0.9 0.91428571 0.92857143 0.94285714 0.95714286 0.97142857 0.98571429 1 1 1 1 1 1
  arc A22 (-7.6109, 0.373) -> (-7.6109, -0.373) centre (0, 0) ccw
  spline S11 degree 5 poles (-7.6109, -0.373) (-7.6061, -0.3765) (-7.5966, -0.3833) (-7.5822, -0.3935) (-7.5631, -0.4069) (-7.5391, -0.4236) (-7.5151, -0.44) (-7.491, -0.4562) (-7.4669, -0.4723) (-7.4428, -0.4882) (-7.4186, -0.5038) (-7.3943, -0.5193) (-7.37, -0.5346) (-7.3457, -0.5497) (-7.3213, -0.5646) (-7.2969, -0.5793) (-7.2725, -0.5938) (-7.248, -0.6081) (-7.2235, -0.6222) (-7.1989, -0.6361) (-7.1743, -0.6498) (-7.1497, -0.6632) (-7.125, -0.6765) (-7.1003, -0.6896) (-7.0756, -0.7025) (-7.0508, -0.7151) (-7.0261, -0.7275) (-7.0012, -0.7398) (-6.9764, -0.7518) (-6.9515, -0.7636) (-6.9267, -0.7752) (-6.9017, -0.7865) (-6.8768, -0.7977) (-6.8519, -0.8086) (-6.8269, -0.8193) (-6.8019, -0.8297) (-6.7769, -0.84) (-6.7519, -0.85) (-6.7268, -0.8598) (-6.7018, -0.8693) (-6.6767, -0.8786) (-6.6516, -0.8877) (-6.6265, -0.8965) (-6.6014, -0.9051) (-6.5763, -0.9134) (-6.5512, -0.9215) (-6.5261, -0.9293) (-6.501, -0.9369) (-6.4759, -0.9442) (-6.4508, -0.9513) (-6.4257, -0.9581) (-6.4006, -0.9646) (-6.3755, -0.9708) (-6.3504, -0.9767) (-6.3253, -0.9823) (-6.3003, -0.9876) (-6.2752, -0.9927) (-6.2502, -0.9975) (-6.2251, -1.002) (-6.2001, -1.0063) (-6.1752, -1.0101) (-6.1502, -1.0135) (-6.1253, -1.0165) (-6.1004, -1.0189) (-6.0756, -1.021) (-6.0508, -1.0228) (-6.026, -1.0244) (-6.0013, -1.0257) (-5.9766, -1.0267) (-5.952, -1.0272) (-5.9275, -1.0267) (-5.908, -1.0253) (-5.8935, -1.0235) (-5.8838, -1.022) (-5.879, -1.0212) knots -1 -1 -1 -1 -1 -1 -0.98571429 -0.97142857 -0.95714286 -0.94285714 -0.92857143 -0.91428571 -0.9 -0.88571429 -0.87142857 -0.85714286 -0.84285714 -0.82857143 -0.81428571 -0.8 -0.78571429 -0.77142857 -0.75714286 -0.74285714 -0.72857143 -0.71428571 -0.7 -0.68571429 -0.67142857 -0.65714286 -0.64285714 -0.62857143 -0.61428571 -0.6 -0.58571429 -0.57142857 -0.55714286 -0.54285714 -0.52857143 -0.51428571 -0.5 -0.48571429 -0.47142857 -0.45714286 -0.44285714 -0.42857143 -0.41428571 -0.4 -0.38571429 -0.37142857 -0.35714286 -0.34285714 -0.32857143 -0.31428571 -0.3 -0.28571429 -0.27142857 -0.25714286 -0.24285714 -0.22857143 -0.21428571 -0.2 -0.18571429 -0.17142857 -0.15714286 -0.14285714 -0.12857143 -0.11428571 -0.1 -0.08571429 -0.07142857 -0.05714286 -0.04285714 -0.02857143 -0.01428571 0 0 0 0 0 0
  line L11 (-5.879, -1.0212) -> (-5.0018, -0.8688)
  arc A23 (-4.772, -1.0239) -> (-5.0018, -0.8688) centre (-4.9675, -1.0659) ccw
  arc A24 (-4.772, -1.0239) -> (-4.4625, -1.9766) centre (0, 0) ccw
  arc A25 (-4.5572, -2.2371) -> (-4.4625, -1.9766) centre (-4.6453, -2.0576) ccw
  line L12 (-4.5572, -2.2371) -> (-5.3565, -2.6294)
  spline S12 degree 5 poles (-5.3565, -2.6294) (-5.3609, -2.6316) (-5.3696, -2.6361) (-5.3824, -2.6432) (-5.3989, -2.6535) (-5.419, -2.6675) (-5.4387, -2.6823) (-5.458, -2.6976) (-5.4773, -2.7133) (-5.4964, -2.7291) (-5.5154, -2.7451) (-5.5343, -2.7614) (-5.5529, -2.778) (-5.5713, -2.7951) (-5.5895, -2.8125) (-5.6075, -2.8303) (-5.6252, -2.8484) (-5.6428, -2.8668) (-5.6602, -2.8854) (-5.6775, -2.9042) (-5.6947, -2.9233) (-5.7117, -2.9425) (-5.7285, -2.9621) (-5.7451, -2.9818) (-5.7616, -3.0018) (-5.7779, -3.0221) (-5.7941, -3.0426) (-5.8101, -3.0633) (-5.826, -3.0842) (-5.8417, -3.1052) (-5.8572, -3.1265) (-5.8727, -3.148) (-5.8879, -3.1697) (-5.903, -3.1916) (-5.918, -3.2137) (-5.9328, -3.2359) (-5.9475, -3.2584) (-5.962, -3.281) (-5.9763, -3.3038) (-5.9905, -3.3268) (-6.0046, -3.3499) (-6.0185, -3.3733) (-6.0323, -3.3968) (-6.0459, -3.4204) (-6.0594, -3.4443) (-6.0727, -3.4683) (-6.0859, -3.4924) (-6.099, -3.5167) (-6.1118, -3.5412) (-6.1246, -3.5658) (-6.1372, -3.5906) (-6.1496, -3.6156) (-6.1619, -3.6407) (-6.1741, -3.6659) (-6.1861, -3.6913) (-6.1979, -3.7168) (-6.2096, -3.7425) (-6.2212, -3.7683) (-6.2326, -3.7943) (-6.2438, -3.8204) (-6.255, -3.8466) (-6.2659, -3.873) (-6.2767, -3.8995) (-6.2874, -3.9261) (-6.2979, -3.9529) (-6.3083, -3.9798) (-6.3185, -4.0069) (-6.3286, -4.034) (-6.3385, -4.0613) (-6.3482, -4.0887) (-6.3579, -4.1163) (-6.3654, -4.1384) (-6.371, -4.1551) (-6.3747, -4.1662) (-6.3766, -4.1718) knots 0 0 0 0 0 0 0.01428571 0.02857143 0.04285714 0.05714286 0.07142857 0.08571429 0.1 0.11428571 0.12857143 0.14285714 0.15714286 0.17142857 0.18571429 0.2 0.21428571 0.22857143 0.24285714 0.25714286 0.27142857 0.28571429 0.3 0.31428571 0.32857143 0.34285714 0.35714286 0.37142857 0.38571429 0.4 0.41428571 0.42857143 0.44285714 0.45714286 0.47142857 0.48571429 0.5 0.51428571 0.52857143 0.54285714 0.55714286 0.57142857 0.58571429 0.6 0.61428571 0.62857143 0.64285714 0.65714286 0.67142857 0.68571429 0.7 0.71428571 0.72857143 0.74285714 0.75714286 0.77142857 0.78571429 0.8 0.81428571 0.82857143 0.84285714 0.85714286 0.87142857 0.88571429 0.9 0.91428571 0.92857143 0.94285714 0.95714286 0.97142857 0.98571429 1 1 1 1 1 1
  arc A26 (-6.3766, -4.1718) -> (-5.938, -4.7754) centre (0, 0) ccw
  spline S13 degree 5 poles (-5.938, -4.7754) (-5.9322, -4.7753) (-5.9204, -4.7752) (-5.9029, -4.775) (-5.8795, -4.7747) (-5.8503, -4.774) (-5.8212, -4.7732) (-5.7922, -4.7722) (-5.7633, -4.7711) (-5.7344, -4.7697) (-5.7056, -4.7682) (-5.6769, -4.7664) (-5.6483, -4.7645) (-5.6197, -4.7624) (-5.5912, -4.7602) (-5.5628, -4.7577) (-5.5345, -4.755) (-5.5063, -4.7522) (-5.4782, -4.7492) (-5.4502, -4.746) (-5.4222, -4.7426) (-5.3944, -4.7391) (-5.3666, -4.7353) (-5.3389, -4.7314) (-5.3114, -4.7272) (-5.2839, -4.7229) (-5.2566, -4.7184) (-5.2293, -4.7137) (-5.2021, -4.7088) (-5.1751, -4.7038) (-5.1481, -4.6985) (-5.1213, -4.6931) (-5.0946, -4.6874) (-5.068, -4.6816) (-5.0415, -4.6755) (-5.0151, -4.6693) (-4.9889, -4.6629) (-4.9628, -4.6563) (-4.9368, -4.6495) (-4.9109, -4.6425) (-4.8851, -4.6353) (-4.8595, -4.6279) (-4.834, -4.6203) (-4.8087, -4.6124) (-4.7835, -4.6044) (-4.7584, -4.5962) (-4.7335, -4.5878) (-4.7088, -4.5791) (-4.6841, -4.5703) (-4.6597, -4.5613) (-4.6354, -4.552) (-4.6112, -4.5425) (-4.5873, -4.5328) (-4.5635, -4.5228) (-4.5399, -4.5126) (-4.5165, -4.5022) (-4.4933, -4.4916) (-4.4702, -4.4807) (-4.4473, -4.4697) (-4.4246, -4.4584) (-4.4021, -4.4468) (-4.3799, -4.4349) (-4.358, -4.4227) (-4.3364, -4.4101) (-4.3151, -4.3972) (-4.294, -4.384) (-4.273, -4.3707) (-4.2522, -4.3573) (-4.2317, -4.3436) (-4.2115, -4.3295) (-4.192, -4.3147) (-4.177, -4.3021) (-4.1663, -4.2922) (-4.1594, -4.2853) (-4.156, -4.2818) knots -1 -1 -1 -1 -1 -1 -0.98571429 -0.97142857 -0.95714286 -0.94285714 -0.92857143 -0.91428571 -0.9 -0.88571429 -0.87142857 -0.85714286 -0.84285714 -0.82857143 -0.81428571 -0.8 -0.78571429 -0.77142857 -0.75714286 -0.74285714 -0.72857143 -0.71428571 -0.7 -0.68571429 -0.67142857 -0.65714286 -0.64285714 -0.62857143 -0.61428571 -0.6 -0.58571429 -0.57142857 -0.55714286 -0.54285714 -0.52857143 -0.51428571 -0.5 -0.48571429 -0.47142857 -0.45714286 -0.44285714 -0.42857143 -0.41428571 -0.4 -0.38571429 -0.37142857 -0.35714286 -0.34285714 -0.32857143 -0.31428571 -0.3 -0.28571429 -0.27142857 -0.25714286 -0.24285714 -0.22857143 -0.21428571 -0.2 -0.18571429 -0.17142857 -0.15714286 -0.14285714 -0.12857143 -0.11428571 -0.1 -0.08571429 -0.07142857 -0.05714286 -0.04285714 -0.02857143 -0.01428571 0 0 0 0 0 0
  line L13 (-4.156, -4.2818) -> (-3.5358, -3.6429)
  arc A27 (-3.2588, -3.6333) -> (-3.5358, -3.6429) centre (-3.3923, -3.7821) ccw
  arc A28 (-3.2588, -3.6333) -> (-2.4484, -4.222) centre (0, 0) ccw
  arc A29 (-2.3719, -4.4885) -> (-2.4484, -4.222) centre (-2.5487, -4.3951) ccw
  line L14 (-2.3719, -4.4885) -> (-2.7879, -5.2757)
  spline S14 degree 5 poles (-2.7879, -5.2757) (-2.7902, -5.28) (-2.7946, -5.2888) (-2.8008, -5.302) (-2.8082, -5.3201) (-2.8162, -5.3433) (-2.8234, -5.3668) (-2.83, -5.3906) (-2.8364, -5.4145) (-2.8426, -5.4386) (-2.8485, -5.4627) (-2.8542, -5.487) (-2.8595, -5.5114) (-2.8644, -5.536) (-2.8689, -5.5608) (-2.8729, -5.5857) (-2.8767, -5.6108) (-2.8801, -5.636) (-2.8832, -5.6613) (-2.8862, -5.6867) (-2.8888, -5.7122) (-2.8912, -5.7378) (-2.8934, -5.7635) (-2.8952, -5.7893) (-2.8968, -5.8151) (-2.8981, -5.8411) (-2.8991, -5.8672) (-2.8999, -5.8933) (-2.9005, -5.9196) (-2.9008, -5.9459) (-2.9009, -5.9722) (-2.9007, -5.9987) (-2.9003, -6.0252) (-2.8997, -6.0518) (-2.8988, -6.0784) (-2.8977, -6.1051) (-2.8964, -6.1319) (-2.8948, -6.1587) (-2.893, -6.1856) (-2.891, -6.2126) (-2.8888, -6.2396) (-2.8863, -6.2666) (-2.8837, -6.2937) (-2.8808, -6.3209) (-2.8777, -6.3481) (-2.8744, -6.3753) (-2.8708, -6.4026) (-2.8671, -6.43) (-2.8631, -6.4574) (-2.8589, -6.4848) (-2.8546, -6.5122) (-2.85, -6.5397) (-2.8452, -6.5672) (-2.8402, -6.5948) (-2.8349, -6.6224) (-2.8295, -6.65) (-2.8239, -6.6777) (-2.8181, -6.7053) (-2.8121, -6.7331) (-2.8058, -6.7608) (-2.7994, -6.7885) (-2.7928, -6.8163) (-2.7859, -6.8441) (-2.7789, -6.872) (-2.7717, -6.8998) (-2.7642, -6.9277) (-2.7566, -6.9555) (-2.7488, -6.9834) (-2.7408, -7.0113) (-2.7325, -7.0392) (-2.7241, -7.0672) (-2.7172, -7.0895) (-2.712, -7.1063) (-2.7085, -7.1175) (-2.7067, -7.1231) knots 0 0 0 0 0 0 0.01428571 0.02857143 0.04285714 0.05714286 0.07142857 0.08571429 0.1 0.11428571 0.12857143 0.14285714 0.15714286 0.17142857 0.18571429 0.2 0.21428571 0.22857143 0.24285714 0.25714286 0.27142857 0.28571429 0.3 0.31428571 0.32857143 0.34285714 0.35714286 0.37142857 0.38571429 0.4 0.41428571 0.42857143 0.44285714 0.45714286 0.47142857 0.48571429 0.5 0.51428571 0.52857143 0.54285714 0.55714286 0.57142857 0.58571429 0.6 0.61428571 0.62857143 0.64285714 0.65714286 0.67142857 0.68571429 0.7 0.71428571 0.72857143 0.74285714 0.75714286 0.77142857 0.78571429 0.8 0.81428571 0.82857143 0.84285714 0.85714286 0.87142857 0.88571429 0.9 0.91428571 0.92857143 0.94285714 0.95714286 0.97142857 0.98571429 1 1 1 1 1 1
  arc A30 (-2.7067, -7.1231) -> (-1.9971, -7.3536) centre (0, 0) ccw
  spline S15 degree 5 poles (-1.9971, -7.3536) (-1.9924, -7.3502) (-1.9829, -7.3432) (-1.9688, -7.3327) (-1.9501, -7.3187) (-1.9269, -7.301) (-1.9038, -7.2833) (-1.8809, -7.2654) (-1.8582, -7.2474) (-1.8357, -7.2294) (-1.8133, -7.2112) (-1.7911, -7.1929) (-1.769, -7.1745) (-1.7471, -7.1561) (-1.7255, -7.1375) (-1.7039, -7.1188) (-1.6826, -7.1) (-1.6614, -7.0812) (-1.6404, -7.0622) (-1.6196, -7.0431) (-1.599, -7.024) (-1.5786, -7.0047) (-1.5583, -6.9854) (-1.5383, -6.9659) (-1.5184, -6.9464) (-1.4987, -6.9267) (-1.4792, -6.907) (-1.4599, -6.8872) (-1.4408, -6.8673) (-1.4219, -6.8473) (-1.4032, -6.8272) (-1.3847, -6.807) (-1.3664, -6.7867) (-1.3483, -6.7664) (-1.3305, -6.7459) (-1.3128, -6.7254) (-1.2953, -6.7048) (-1.2781, -6.6841) (-1.261, -6.6633) (-1.2442, -6.6424) (-1.2276, -6.6214) (-1.2112, -6.6004) (-1.1951, -6.5792) (-1.1792, -6.558) (-1.1635, -6.5367) (-1.1481, -6.5153) (-1.1329, -6.4939) (-1.1179, -6.4723) (-1.1032, -6.4507) (-1.0887, -6.429) (-1.0745, -6.4072) (-1.0605, -6.3854) (-1.0469, -6.3634) (-1.0335, -6.3414) (-1.0204, -6.3193) (-1.0076, -6.2971) (-0.995, -6.2748) (-0.9827, -6.2525) (-0.9707, -6.2301) (-0.9589, -6.2076) (-0.9476, -6.1851) (-0.9366, -6.1624) (-0.9261, -6.1396) (-0.9161, -6.1167) (-0.9064, -6.0937) (-0.897, -6.0707) (-0.8879, -6.0476) (-0.879, -6.0245) (-0.8704, -6.0014) (-0.8623, -5.9781) (-0.8552, -5.9547) (-0.8506, -5.9357) (-0.8478, -5.9213) (-0.8462, -5.9117) (-0.8455, -5.9068) knots -1 -1 -1 -1 -1 -1 -0.98571429 -0.97142857 -0.95714286 -0.94285714 -0.92857143 -0.91428571 -0.9 -0.88571429 -0.87142857 -0.85714286 -0.84285714 -0.82857143 -0.81428571 -0.8 -0.78571429 -0.77142857 -0.75714286 -0.74285714 -0.72857143 -0.71428571 -0.7 -0.68571429 -0.67142857 -0.65714286 -0.64285714 -0.62857143 -0.61428571 -0.6 -0.58571429 -0.57142857 -0.55714286 -0.54285714 -0.52857143 -0.51428571 -0.5 -0.48571429 -0.47142857 -0.45714286 -0.44285714 -0.42857143 -0.41428571 -0.4 -0.38571429 -0.37142857 -0.35714286 -0.34285714 -0.32857143 -0.31428571 -0.3 -0.28571429 -0.27142857 -0.25714286 -0.24285714 -0.22857143 -0.21428571 -0.2 -0.18571429 -0.17142857 -0.15714286 -0.14285714 -0.12857143 -0.11428571 -0.1 -0.08571429 -0.07142857 -0.05714286 -0.04285714 -0.02857143 -0.01428571 0 0 0 0 0 0
  line L15 (-0.8455, -5.9068) -> (-0.7193, -5.0254)
  arc A31 (-0.5008, -4.8548) -> (-0.7193, -5.0254) centre (-0.5214, -5.0538) ccw
  arc A32 (-0.5008, -4.8548) -> (0.5008, -4.8548) centre (0, 0) ccw
  arc A33 (0.7193, -5.0254) -> (0.5008, -4.8548) centre (0.5214, -5.0538) ccw
  line L16 (0.7193, -5.0254) -> (0.8455, -5.9068)
  spline S16 degree 5 poles (0.8455, -5.9068) (0.8462, -5.9117) (0.8478, -5.9213) (0.8506, -5.9357) (0.8552, -5.9547) (0.8623, -5.9781) (0.8704, -6.0014) (0.879, -6.0245) (0.8879, -6.0476) (0.897, -6.0707) (0.9064, -6.0937) (0.9161, -6.1167) (0.9261, -6.1396) (0.9366, -6.1624) (0.9476, -6.1851) (0.9589, -6.2076) (0.9707, -6.2301) (0.9827, -6.2525) (0.995, -6.2748) (1.0076, -6.2971) (1.0204, -6.3193) (1.0335, -6.3414) (1.0469, -6.3634) (1.0605, -6.3854) (1.0745, -6.4072) (1.0887, -6.429) (1.1032, -6.4507) (1.1179, -6.4723) (1.1329, -6.4939) (1.1481, -6.5153) (1.1635, -6.5367) (1.1792, -6.558) (1.1951, -6.5792) (1.2112, -6.6004) (1.2276, -6.6214) (1.2442, -6.6424) (1.261, -6.6633) (1.2781, -6.6841) (1.2953, -6.7048) (1.3128, -6.7254) (1.3305, -6.7459) (1.3483, -6.7664) (1.3664, -6.7867) (1.3847, -6.807) (1.4032, -6.8272) (1.4219, -6.8473) (1.4408, -6.8673) (1.4599, -6.8872) (1.4792, -6.907) (1.4987, -6.9267) (1.5184, -6.9464) (1.5383, -6.9659) (1.5583, -6.9854) (1.5786, -7.0047) (1.599, -7.024) (1.6196, -7.0431) (1.6404, -7.0622) (1.6614, -7.0812) (1.6826, -7.1) (1.7039, -7.1188) (1.7255, -7.1375) (1.7471, -7.1561) (1.769, -7.1745) (1.7911, -7.1929) (1.8133, -7.2112) (1.8357, -7.2294) (1.8582, -7.2474) (1.8809, -7.2654) (1.9038, -7.2833) (1.9269, -7.301) (1.9501, -7.3187) (1.9688, -7.3327) (1.9829, -7.3432) (1.9924, -7.3502) (1.9971, -7.3536) knots 0 0 0 0 0 0 0.01428571 0.02857143 0.04285714 0.05714286 0.07142857 0.08571429 0.1 0.11428571 0.12857143 0.14285714 0.15714286 0.17142857 0.18571429 0.2 0.21428571 0.22857143 0.24285714 0.25714286 0.27142857 0.28571429 0.3 0.31428571 0.32857143 0.34285714 0.35714286 0.37142857 0.38571429 0.4 0.41428571 0.42857143 0.44285714 0.45714286 0.47142857 0.48571429 0.5 0.51428571 0.52857143 0.54285714 0.55714286 0.57142857 0.58571429 0.6 0.61428571 0.62857143 0.64285714 0.65714286 0.67142857 0.68571429 0.7 0.71428571 0.72857143 0.74285714 0.75714286 0.77142857 0.78571429 0.8 0.81428571 0.82857143 0.84285714 0.85714286 0.87142857 0.88571429 0.9 0.91428571 0.92857143 0.94285714 0.95714286 0.97142857 0.98571429 1 1 1 1 1 1
  arc A34 (1.9971, -7.3536) -> (2.7067, -7.1231) centre (0, 0) ccw
  spline S17 degree 5 poles (2.7067, -7.1231) (2.7085, -7.1175) (2.712, -7.1063) (2.7172, -7.0895) (2.7241, -7.0672) (2.7325, -7.0392) (2.7408, -7.0113) (2.7488, -6.9834) (2.7566, -6.9555) (2.7642, -6.9277) (2.7717, -6.8998) (2.7789, -6.872) (2.7859, -6.8441) (2.7928, -6.8163) (2.7994, -6.7885) (2.8058, -6.7608) (2.8121, -6.7331) (2.8181, -6.7053) (2.8239, -6.6777) (2.8295, -6.65) (2.8349, -6.6224) (2.8402, -6.5948) (2.8452, -6.5672) (2.85, -6.5397) (2.8546, -6.5122) (2.8589, -6.4848) (2.8631, -6.4574) (2.8671, -6.43) (2.8708, -6.4026) (2.8744, -6.3753) (2.8777, -6.3481) (2.8808, -6.3209) (2.8837, -6.2937) (2.8863, -6.2666) (2.8888, -6.2396) (2.891, -6.2126) (2.893, -6.1856) (2.8948, -6.1587) (2.8964, -6.1319) (2.8977, -6.1051) (2.8988, -6.0784) (2.8997, -6.0518) (2.9003, -6.0252) (2.9007, -5.9987) (2.9009, -5.9722) (2.9008, -5.9459) (2.9005, -5.9196) (2.8999, -5.8933) (2.8991, -5.8672) (2.8981, -5.8411) (2.8968, -5.8151) (2.8952, -5.7893) (2.8934, -5.7635) (2.8912, -5.7378) (2.8888, -5.7122) (2.8862, -5.6867) (2.8832, -5.6613) (2.8801, -5.636) (2.8767, -5.6108) (2.8729, -5.5857) (2.8689, -5.5608) (2.8644, -5.536) (2.8595, -5.5114) (2.8542, -5.487) (2.8485, -5.4627) (2.8426, -5.4386) (2.8364, -5.4145) (2.83, -5.3906) (2.8234, -5.3668) (2.8162, -5.3433) (2.8082, -5.3201) (2.8008, -5.302) (2.7946, -5.2888) (2.7902, -5.28) (2.7879, -5.2757) knots -1 -1 -1 -1 -1 -1 -0.98571429 -0.97142857 -0.95714286 -0.94285714 -0.92857143 -0.91428571 -0.9 -0.88571429 -0.87142857 -0.85714286 -0.84285714 -0.82857143 -0.81428571 -0.8 -0.78571429 -0.77142857 -0.75714286 -0.74285714 -0.72857143 -0.71428571 -0.7 -0.68571429 -0.67142857 -0.65714286 -0.64285714 -0.62857143 -0.61428571 -0.6 -0.58571429 -0.57142857 -0.55714286 -0.54285714 -0.52857143 -0.51428571 -0.5 -0.48571429 -0.47142857 -0.45714286 -0.44285714 -0.42857143 -0.41428571 -0.4 -0.38571429 -0.37142857 -0.35714286 -0.34285714 -0.32857143 -0.31428571 -0.3 -0.28571429 -0.27142857 -0.25714286 -0.24285714 -0.22857143 -0.21428571 -0.2 -0.18571429 -0.17142857 -0.15714286 -0.14285714 -0.12857143 -0.11428571 -0.1 -0.08571429 -0.07142857 -0.05714286 -0.04285714 -0.02857143 -0.01428571 0 0 0 0 0 0
  line L17 (2.7879, -5.2757) -> (2.3719, -4.4885)
  arc A35 (2.4484, -4.222) -> (2.3719, -4.4885) centre (2.5487, -4.3951) ccw
  arc A36 (2.4484, -4.222) -> (3.2588, -3.6333) centre (0, 0) ccw
  arc A37 (3.5358, -3.6429) -> (3.2588, -3.6333) centre (3.3923, -3.7821) ccw
  line L18 (3.5358, -3.6429) -> (4.156, -4.2818)